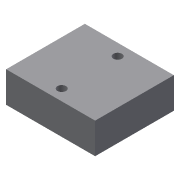
# Autodesk Inventor part: +5V Regulator
Saved by Autodesk Inventor 2013 (Build 170138000, 138)
## iProperties
Created: 2014-01-15
Part Number: +5V Regulator
Material: Generic
Document SubType Name: Modeling
Designer: aldalziel
Density: 1.57913 g/cm^3
Mass: 136.985 g
Surface Area: 141.918 cm^2
Volume: 86.7473 cm^3
Author: aldalziel
Autodesk Inventor part; units mm, degrees
ref_plane "YZ Plane" through (0, 0, 0) normal (1, 0, 0) x (0, 1, 0)
ref_plane "XZ Plane" through (0, 0, 0) normal (0, 1, 0) x (-1, 0, 0)
ref_plane "XY Plane" through (0, 0, 0) normal (0, 0, 1) x (1, 0, 0)
sketch "Sketch1" plane through (0, 0, 0) normal (0, 0, 1) x (1, 0, 0)
  line L0 (0, 0) -> (66.04, 0)
  line L1 (66.04, 0) -> (66.04, 58.42)
  line L2 (66.04, 58.42) -> (0, 58.42)
  line L3 (0, 58.42) -> (0, 0)
  dimension "d0" = 66.04
  dimension "d1" = 58.42
  constraints: 8 end point, 2 parallel, 1 horizontal, 1 perpendicular
  measures "d0" distance of L2.end L1.end
  measures "d1" distance of L1.end L0.end
extrude "Extrusion1" add sketch "Sketch1" along normal blind 22.86
sketch "Sketch2" plane through (0, 0, 22.86) normal (0, 0, 1) x (1, 0, 0)
  line L0 (0, 0) -> (66.04, 0) projected
  point P0 (33.02, 49.7501)
  point P1 (33.02, 8.221)
  point P2 (33.02, 0)
  point P3 (33.02, 0)
  constraints: 2 midpoint, 2 vertical alignment
hole "Hole1" at (33.02, 49.7501, 22.86) at (33.02, 8.221, 22.86) direction (0, 0, -1) diameter 6.35 end through all
body "Solid1"
